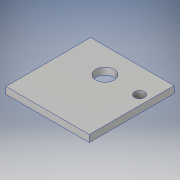
# Autodesk Inventor part: Marco_frontal
Saved by Autodesk Inventor 2019 (Build 230136000, 136)
## iProperties
Created: 2019-11-14
Part Number: Marco_frontal
Material: Aluminum 6061
Document SubType Name: Modeling
Designer: Domenico
Density: 2.7 g/cm^3
Appearance: Aluminum - Flat
Mass: 275.525 g
Surface Area: 277.471 cm^2
Volume: 102.046 cm^3
d3: 12.300 mm
Author: Domenico
Autodesk Inventor part; units mm, degrees
ref_plane "YZ Plane" through (0, 0, 0) normal (1, 0, 0) x (0, 1, 0)
ref_plane "XZ Plane" through (0, 0, 0) normal (0, 1, 0) x (-1, 0, 0)
ref_plane "XY Plane" through (0, 0, 0) normal (0, 0, 1) x (1, 0, 0)
sketch "Sketch1" plane through (0, 0, 0) normal (0, 1, 0) x (-1, 0, 0)
  line L0 (0, 0) -> (108.6, 0)
  line L1 (108.6, 0) -> (108.6, -110.4)
  line L2 (108.6, -110.4) -> (0, -110.4)
  line L3 (0, -110.4) -> (0, 0)
  circle A0 centre (12.3, -77.7) radius 6.5
  circle A1 centre (57.3, -77.7) radius 12
  dimension "d0" = 108.6
  dimension "d1" = 110.4
  dimension "d2" = 13
  dimension "d3" = 12.3
  dimension "d4" = 32.7
  dimension "d5" = 24
  dimension "d6" = 45
  constraints: 8 end point, 2 centre point, 2 parallel, 1 coincident, 1 horizontal, 1 horizontal alignment, 1 perpendicular
  measures "d0" distance of L1.end L2.end
  measures "d1" distance between parallel lines of L2 L0
  measures "d2" diameter of A0
  measures "d3" distance from line of L3 A0.centre
  measures "d4" distance from line of L2 A0.centre
  measures "d5" diameter of A1
  measures "d6" distance of A0.centre A1.centre
extrude "Extrusion1" add sketch "Sketch1" along normal blind 9
body "Solid1"
